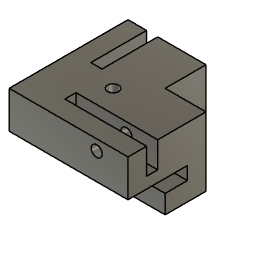
CarrierWallsv1 (Autodesk Fusion 360 archive; units mm, degrees)
design "hammockHolder"
Autodesk Fusion 360 part; units mm, degrees
sketch "Sketch1" plane through (0, 0, 0) normal (0, 0, 1) x (1, 0, 0)
  line L0 (0, 0) -> (11, 0)
  line L1 (11, 0) -> (11, 22)
  line L2 (11, 22) -> (0, 22)
  line L3 (0, 22) -> (0, 0)
  line L4 (11, 0) -> (22, 0)
  line L5 (22, 0) -> (22, 11)
  line L6 (22, 11) -> (11, 11)
  line L7 (11, 11) -> (11, 0)
  dimension "d1" = 11
  dimension "d2" = 22
  dimension "d3" = 11
  dimension "d4" = 11
  constraint horizontal L0
  constraint vertical L1
  constraint horizontal L2
  constraint vertical L3
  constraint coincident L0.start L3.end
  constraint horizontal L4
  constraint vertical L5
  constraint horizontal L6
  constraint vertical L7
  measures "d1" distance of L0.start L0.end
  measures "d2" distance of L0.start L2.end
  measures "d3" distance of L0.end L4.end
  measures "d4" distance of L0.end L6.end
extrude "Extrude1" add sketch "Sketch1" along normal blind 5
sketch "Sketch2" plane through (0, 0, 5) normal (0, 0, 1) x (-1, 0, 0)
  line L0 (-22, -11) -> (-11, -11)
  line L1 (-11, -11) -> (-11, -22)
  line L2 (-11, -22) -> (0, -22)
  line L3 (0, -22) -> (0, 0)
  line L4 (0, 0) -> (-22, 0)
  line L5 (-22, 0) -> (-22, -11)
  line L6 (-22, -11) -> (-5.9353, -11)
  line L7 (-5.9353, -11) -> (-5.9353, -5.9846)
  line L8 (-5.9353, -5.9846) -> (-22, -5.9846)
  line L9 (-22, -5.9846) -> (-22, -11)
  line L10 (-5.9353, -22) -> (-11, -22)
  line L11 (-11, -22) -> (-11, -11)
  line L12 (-11, -11) -> (-5.9353, -11)
  line L13 (-5.9353, -11) -> (-5.9353, -22)
  constraint horizontal L6
  constraint vertical L7
  constraint horizontal L8
  constraint vertical L9
  constraint coincident L0.start L5.end
  constraint horizontal L10
  constraint vertical L11
  constraint horizontal L12
  constraint vertical L13
  constraint coincident L0.end L1.start
  constraint coincident L2 L10.start
extrude "Extrude2" add sketch "Sketch2" along normal blind 3.5 contours L0 L5 L6 L7 L8 L9 L12 | L1 L2 L6 L10 L11 L12 L13
sketch "Sketch3" plane through (0, 0, 8.5) normal (0, 0, 1) x (-1, 0, 0)
  line L0 (-5.9353, -5.9846) -> (-22, -5.9846)
  line L1 (-22, -5.9846) -> (-22, -11)
  line L2 (-22, -11) -> (-11, -11)
  line L3 (-11, -11) -> (-11, -22)
  line L4 (-11, -22) -> (-5.9353, -22)
  line L5 (-5.9353, -22) -> (-5.9353, -5.9846)
  line L6 (0, -22) -> (-11, -22)
  line L7 (-11, -22) -> (-11, 0)
  line L8 (-11, 0) -> (0, 0)
  line L9 (0, 0) -> (0, -22)
  line L10 (-11, -11) -> (-22, -11)
  line L11 (-22, -11) -> (-22, 0)
  line L12 (-22, 0) -> (-11, 0)
  line L13 (-11, 0) -> (-11, -11)
  constraint horizontal L6
  constraint vertical L7
  constraint horizontal L8
  constraint vertical L9
  constraint horizontal L10
  constraint vertical L11
  constraint horizontal L12
  constraint vertical L13
  constraint coincident L2.end L3.start
extrude "Extrude3" add sketch "Sketch3" along normal blind 10
sketch "Sketch4" plane through (0, 0, 18.5) normal (0, 0, 1) x (-1, 0, 0)
  line L0 (-22, 0) -> (-22, -11)
  line L1 (-22, -11) -> (-11, -11)
  line L2 (-11, -11) -> (-11, -22)
  line L3 (-11, -22) -> (0, -22)
  line L4 (0, -22) -> (0, 0)
  line L5 (0, 0) -> (-22, 0)
  circle A0 centre (-4, -4) radius 1.5
  dimension "d11" = 3
  measures "d11" diameter of A0
extrude "Extrude4" cut sketch "Sketch4" against normal blind 17 contours A0
sketch "Sketch5" plane through (0, 0, 18.5) normal (0, 0, 1) x (-1, 0, 0)
  circle A0 centre (-4, -4) radius 1.5
  line L0 (-22, 0) -> (-22, -11)
  line L1 (-22, -11) -> (-11, -11)
  line L2 (-11, -11) -> (-11, -22)
  line L3 (-11, -22) -> (0, -22)
  line L4 (0, -22) -> (0, 0)
  line L5 (0, 0) -> (-22, 0)
  line L6 (-11, -16.4954) -> (0, -16.4954) construction
  line L7 (-4, -22) -> (-7, -22)
  line L8 (-7, -22) -> (-7, -10.9908)
  line L9 (-7, -10.9908) -> (-4, -10.9908)
  line L10 (-4, -10.9908) -> (-4, -22)
  line L11 (-4, -22) -> (-7, -10.9908) construction
  line L12 (-7, -22) -> (-4, -10.9908) construction
  line L13 (-11, -11) -> (-11, 0) construction
  line L14 (-11, -4) -> (-22.0395, -4)
  line L15 (-22.0395, -4) -> (-22.0395, -7)
  line L16 (-22.0395, -7) -> (-11, -7)
  line L17 (-11, -7) -> (-11, -4)
  line L18 (-11, -4) -> (-22.0395, -7) construction
  line L19 (-22.0395, -4) -> (-11, -7) construction
  point P0 (-5.5, -16.4954)
  point P1 (-16.5198, -5.5)
  constraint coincident L2 L6.start
  constraint coincident L4 L6.end
  constraint perpendicular L4 L6
  constraint horizontal L7
  constraint perpendicular L7 L8
  constraint parallel L7 L9
  constraint parallel L8 L10
  constraint coincident L11 P0
  constraint coincident L12 P0
  constraint coincident L3 L7.start
  constraint midpoint L6 P0
  constraint coincident L1.end L2.start
  constraint midpoint L5 L13.end
  constraint horizontal L14
  constraint perpendicular L14 L15
  constraint parallel L14 L16
  constraint parallel L15 L17
  constraint coincident L18 P1
  constraint coincident L19 P1
  constraint coincident L13 L14.start
extrude "Extrude6" add 1 faces at (14.6667, 0, 15.1667) along direction (0, -1, 0) blind 10
extrude "Extrude7" add 1 faces at (0, 0.6667, 15.1667) along direction (-1, 0, 0) blind 10
sketch "Sketch6" plane through (0, 0, 18.5) normal (0, 0, 1) x (-1, 0, 0)
  circle A0 centre (-4, -4) radius 1.5
  line L0 (-22, 10) -> (-22, -11)
  line L1 (-22, -11) -> (-11, -11)
  line L2 (-11, -11) -> (-11, -22)
  line L3 (-11, -22) -> (10, -22)
  line L4 (10, -22) -> (10, 10)
  line L5 (10, 10) -> (-22, 10)
  line L6 (5, -22) -> (2, -22)
  line L7 (2, -22) -> (2, -7)
  line L8 (2, -7) -> (5, -7)
  line L9 (5, -7) -> (5, -22)
  line L10 (-18.4665, 10) -> (-18.4665, 5) construction
  line L11 (-22, 5) -> (0, 5)
  line L12 (0, 5) -> (0, 2)
  line L13 (0, 2) -> (-22, 2)
  line L14 (-22, 2) -> (-22, 5)
  dimension "d20" = 3
  dimension "d21" = 15
  dimension "d22" = 22
  dimension "d23" = 3
  constraint horizontal L6
  constraint vertical L7
  constraint horizontal L8
  constraint vertical L9
  constraint coincident L3 L6.start
  constraint coincident L5 L10.start
  constraint perpendicular L5 L10
  constraint horizontal L11
  constraint vertical L12
  constraint horizontal L13
  constraint vertical L14
  constraint coincident L0 L11.start
  measures "d20" distance of L6.start L6.end
  measures "d21" distance of L6.start L8.end
  measures "d22" distance of L11.start L11.end
  measures "d23" distance of L11.start L13.end
extrude "Extrude8" cut sketch "Sketch6" against normal blind 7 contours L0 L11 L12 L13 L14 | L3 L6 L7 L8 L9
sketch "Sketch7" plane through (0, -10, 0) normal (0, -1, 0) x (1, 0, 0)
  line L0 (-10, 8.5) -> (22, 8.5)
  line L1 (22, 8.5) -> (22, 18.5)
  line L2 (22, 18.5) -> (-10, 18.5)
  line L3 (-10, 18.5) -> (-10, 8.5)
  circle A0 centre (13.5731, 15.6473) radius 1.5
  dimension "d26" = 3
  measures "d26" diameter of A0
extrude "Extrude9" cut sketch "Sketch7" against normal blind 21 contours A0
